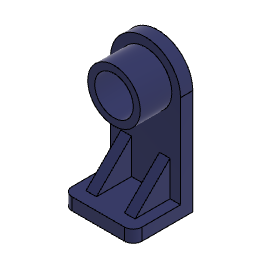
Figure-4 (Autodesk Fusion 360 design; units mm, degrees)
Autodesk Fusion 360 part; units mm, degrees
sketch "Sketch1" plane through (0, 0, 0) normal (0, 0, 1) x (1, 0, 0)
  line L0 (20, 17) -> (-20, 17)
  line L1 (-20, 17) -> (-20, -17)
  line L2 (-20, -17) -> (20, -17)
  line L3 (20, -17) -> (20, 17)
  line L4 (20, 17) -> (-20, -17) construction
  line L5 (-20, 17) -> (20, -17) construction
  dimension "d1" = 40
  dimension "d2" = 34
  constraint horizontal L0
  constraint perpendicular L0 L1
  constraint parallel L0 L2
  constraint parallel L1 L3
  constraint coincident L4 origin
  constraint coincident L5 origin
  measures "d1" distance of L1.end L2.end
  measures "d2" distance of L0.end L1.end
extrude "Extrude1" add sketch "Sketch1" along normal blind 7
fillet "Fillet1" radius 5 2 edges at (20, -17, 3.5) (-20, -17, 3.5)
sketch "Sketch2" plane through (0, 0, 0) normal (0, 1, 0) x (1, 0, 0)
  line L0 (20, 0, 17) -> (-20, 0, 17)
  line L1 (-20, 0, 17) -> (-20, -60, 17)
  line L2 (-20, -60, 17) -> (20, -60, 17)
  line L3 (20, -60, 17) -> (20, 0, 17)
  point P0 (20, 0)
  dimension "d7" = 40
  dimension "d8" = 60
extrude "Extrude2" add sketch "Sketch2" against normal blind 7 contours L0 L1 L2 L3 in plane through (0, 17, 0) normal (0, 1, 0)
sketch "Sketch3" plane through (0, 0, 0) normal (0, 1, 0) x (1, 0, 0)
  circle A0 through (11, -60, 10) (-5.5, -50.4737, 10) (-5.5, -69.5263, 10)
  line L0 (20, -60, 10) -> (-20, -60, 10)
  circle A1 through (15, -60, 10) (-7.5, -47.0096, 10) (-7.5, -72.9904, 10)
  line L1 (20, -60, 17) -> (-20, -60, 17)
  line L2 (-20, -60, 17) -> (-20, -80, 17)
  line L3 (-20, -80, 17) -> (20, -80, 17)
  line L4 (20, -80, 17) -> (20, -60, 17)
  point P0 (20, -60)
  dimension "d11" = 22
  dimension "d12" = 30
  dimension "d13" = 40
  dimension "d14" = 20
extrude "Extrude3" add sketch "Sketch3" against normal blind 7 contours L1 L2 L3 L4 in plane through (0, 17, 0) normal (0, 1, 0)
fillet "Fillet2" radius 20 2 edges at (20, 13.5, 80) (-20, 13.5, 80)
extrude "Extrude4" add sketch "Sketch3" against normal blind 18 contours A0 L0 A1 | A0 L0 A1 in plane through (0, 10, 0) normal (0, 1, 0)
extrude "Extrude5" cut sketch "Sketch3" along normal through all contours A0 L0 | A0 L0 in plane through (0, 10, 0) normal (0, 1, 0)
sketch "Sketch6" plane through (0, 0, 0) normal (0, 0, 1) x (1, 0, 0)
  line L0 (20, 10, 7) -> (-20, 10, 7)
  line L1 (14, 10, 7) -> (14, -10, 7)
  line L2 (20, -12, 7) -> (20, 10, 7)
  line L3 (14, 10, 7) -> (14, 10, 27)
  line L4 (14, 10, 27) -> (14, -10, 7)
  line L5 (-14, 10, 7) -> (-14, -10, 7)
  line L6 (-20, 10, 7) -> (-20, -12, 7)
  line L7 (-14, 10, 7) -> (-14, 10, 27)
  line L8 (-14, 10, 27) -> (-14, -10, 7)
  dimension "d22" = 20
  dimension "d23" = 6
  dimension "d24" = 20
  dimension "d25" = 20
  dimension "d26" = 6
  dimension "d27" = 20
extrude "Extrude6" add sketch "Sketch6" along normal blind 6 contours L5 L7 L8 in plane through (-14, 0, 0) normal (1, 0, 0)
extrude "Extrude7" add sketch "Sketch6" against normal blind 6 contours L1 L3 L4 in plane through (14, 0, 0) normal (1, 0, 0)
